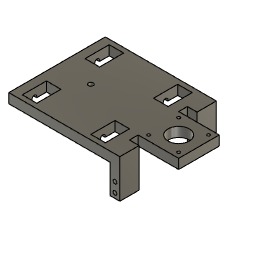
maturita3 v7-asi už konečne final verze (Autodesk Fusion 360 design; units mm, degrees)
Autodesk Fusion 360 part; units mm, degrees
note: some values were not read from the file. Set by a fixed rule: which sketch regions a step uses.
sketch "Sketch1" plane through (0, 0, 0) normal (0, 0, 1) x (1, 0, 0)
  line L0 (0, 0) -> (105, 0)
  line L1 (105, 0) -> (105, 29)
  line L2 (105, 29) -> (147, 29)
  line L3 (147, 29) -> (147, 71)
  line L4 (147, 71) -> (105, 71)
  line L5 (105, 71) -> (105, 100)
  line L6 (105, 100) -> (0, 100)
  line L7 (0, 100) -> (0, 0)
  dimension "d1" = 105
  dimension "d2" = 29
  dimension "d3" = 42
  dimension "d4" = 42
  dimension "d5" = 29
  dimension "d35" = 105
  constraint coincident L0.start L7.end
  constraint horizontal L0
  constraint perpendicular L0 L1
  constraint perpendicular L1 L2
  constraint perpendicular L2 L3
  constraint perpendicular L1 L4
  constraint perpendicular L4 L5
  constraint perpendicular L5 L6
  constraint perpendicular L6 L7
  measures "d1" distance of L0.start L0.end
  measures "d2" distance of L0.end L1.end
  measures "d3" distance of L1.end L2.end
  measures "d4" distance of L2.end L3.end
  measures "d5" distance of L4.end L5.end
  measures "d35" distance of L5.end L6.end
extrude "Extrude1" add sketch "Sketch1" along normal blind 10
sketch "Sketch2" plane through (0, 0, 10) normal (0, 0, 1) x (-1, 0, 0)
  line L0 (0, -100) -> (0, 0)
  line L1 (0, 0) -> (-105, 0)
  line L2 (-105, 0) -> (-105, -29)
  line L3 (-105, -29) -> (-147, -29)
  line L4 (-147, -29) -> (-147, -71)
  line L5 (-147, -71) -> (-105, -71)
  line L6 (-105, -71) -> (-105, -100)
  line L7 (-105, -100) -> (0, -100)
  line L8 (-147, -71) -> (-141.5, -71)
  line L9 (-141.5, -71) -> (-141.5, -65.5)
  line L10 (-141.5, -65.5) -> (-110.5, -65.5)
  line L11 (-110.5, -65.5) -> (-110.5, -34.5)
  line L12 (-110.5, -34.5) -> (-141.5, -34.5)
  line L13 (-141.5, -34.5) -> (-141.5, -65.5)
  dimension "d8" = 5.5
  dimension "d9" = 5.5
  dimension "d10" = 31
  dimension "d11" = 31
  constraint coincident L4.end L5.start
  constraint perpendicular L4 L8
  constraint perpendicular L8 L9
  constraint horizontal L10
  constraint vertical L11
  constraint horizontal L12
  constraint vertical L13
  measures "d8" distance of L4.end L8.end
  measures "d9" distance of L8.end L9.end
  measures "d10" distance of L9.end L10.end
  measures "d11" distance of L9.end L12.end
hole "Hole1" at (110.5, 65.5, 10) at (110.5, 34.5, 10) at (141.5, 34.5, 10) at (141.5, 65.5, 10) direction (0, 0, -1) diameter 3 depth 10 tip angle 180
sketch "Sketch3" plane through (0, 0, 10) normal (0, 0, 1) x (-1, 0, 0)
  circle A0 centre (-141.5, -34.5) radius 1.5
  circle A1 centre (-110.5, -65.5) radius 1.5
  circle A2 centre (-110.5, -34.5) radius 1.5
  circle A3 centre (-141.5, -65.5) radius 1.5
  line L0 (0, -100) -> (0, 0)
  line L1 (0, 0) -> (-105, 0)
  line L2 (-105, 0) -> (-105, -29)
  line L3 (-105, -29) -> (-147, -29)
  line L4 (-147, -29) -> (-147, -71)
  line L5 (-147, -71) -> (-105, -71)
  line L6 (-105, -71) -> (-105, -100)
  line L7 (-105, -100) -> (0, -100)
  line L8 (0, -50) -> (-35, -50)
  circle A4 centre (-35, -50) radius 2.5
  circle A5 centre (-35, -50) radius 5
  dimension "d15" = 5
  dimension "d16" = 10
  dimension "d36" = 35
  constraint midpoint L0 L8.start
  constraint perpendicular L0 L8
  constraint coincident L8.end A4.centre
  measures "d15" diameter of A4
  measures "d16" diameter of A5
  measures "d36" distance of L8.start L8.end
extrude "Extrude2" cut sketch "Sketch3" against normal up to surface (10 mm away) contours A4
extrude "Extrude3" add sketch "Sketch3" along normal blind 1 contours A5
extrude "Extrude4" add 1 faces at (30.8519, 50.2484, 11) along direction (0, 0, -1) blind 20
sketch "Sketch4" plane through (0, 0, -9) normal (0, 0, -1) x (1, 0, 0)
  circle A0 centre (35, -50) radius 2.5
  circle A1 centre (35, -50) radius 5
  circle A2 centre (35, -50) radius 5
  constraint concentric A0 A2
extrude "Extrude5" add sketch "Sketch4" against normal blind 2 contours A0
sketch "Sketch5" plane through (0, 0, 10) normal (0, 0, 1) x (-1, 0, 0)
  line L0 (-115, -100) -> (-95, -100)
  line L1 (-95, -100) -> (-95, -95)
  line L2 (-95, -95) -> (-80, -95)
  line L3 (-80, -95) -> (-80, -70)
  line L4 (-80, -70) -> (-95, -70)
  line L5 (-95, -70) -> (-95, -95)
  dimension "d25" = 20
  dimension "d26" = 5
  dimension "d27" = 15
  dimension "d28" = 25
  constraint horizontal L0
  constraint perpendicular L0 L1
  constraint horizontal L2
  constraint vertical L3
  constraint horizontal L4
  constraint vertical L5
  measures "d25" distance of L0.start L0.end
  measures "d26" distance of L0.end L1.end
  measures "d27" distance of L1.end L2.end
  measures "d28" distance of L1.end L4.end
extrude "Extrude6" cut sketch "Sketch5" against normal blind 10
pattern_linear "R-Pattern1" count 2 spacing 65 along (0, -1, 0) count 2 spacing 71 along (-1, 0, 0) of "Extrude6"
sketch "Sketch6" plane through (0, 0, 10) normal (0, 0, 1) x (-1, 0, 0)
  line L0 (-9, -30) -> (-24, -30)
  line L1 (-24, -30) -> (-24, -5)
  line L2 (-24, -5) -> (-9, -5)
  line L3 (-9, -5) -> (-9, -30)
  line L4 (-9, -95) -> (-24, -95)
  line L5 (-24, -95) -> (-24, -70)
  line L6 (-24, -70) -> (-9, -70)
  line L7 (-9, -70) -> (-9, -95)
  line L8 (-80, -30) -> (-95, -30)
  line L9 (-95, -30) -> (-95, -5)
  line L10 (-95, -5) -> (-80, -5)
  line L11 (-80, -5) -> (-80, -30)
  line L12 (-80, -95) -> (-95, -95)
  line L13 (-95, -95) -> (-95, -70)
  line L14 (-95, -70) -> (-80, -70)
  line L15 (-80, -70) -> (-80, -95)
  circle A0 centre (-35, -50) radius 5
  circle A1 centre (-141.5, -34.5) radius 1.5
  circle A2 centre (-110.5, -65.5) radius 1.5
  circle A3 centre (-110.5, -34.5) radius 1.5
  circle A4 centre (-141.5, -65.5) radius 1.5
  line L16 (0, -100) -> (0, 0)
  line L17 (0, 0) -> (-105, 0)
  line L18 (-105, 0) -> (-105, -29)
  line L19 (-105, -29) -> (-147, -29)
  line L20 (-147, -29) -> (-147, -71)
  line L21 (-147, -71) -> (-105, -71)
  line L22 (-105, -71) -> (-105, -100)
  line L23 (-105, -100) -> (0, -100)
  line L24 (-147, -50) -> (-126, -50)
  constraint midpoint L20 L24.start
  constraint perpendicular L20 L24
hole "Hole2" at (126, 50, 10) direction (0, 0, -1) diameter 22 depth 10 tip angle 180
sketch "Sketch7" plane through (0, 0, 0) normal (0, 0, -1) x (1, 0, 0)
  circle A0 centre (126, -50) radius 11
  line L0 (24, -30) -> (9, -30)
  line L1 (9, -30) -> (9, -5)
  line L2 (9, -5) -> (24, -5)
  line L3 (24, -5) -> (24, -30)
  line L4 (24, -95) -> (9, -95)
  line L5 (9, -95) -> (9, -70)
  line L6 (9, -70) -> (24, -70)
  line L7 (24, -70) -> (24, -95)
  line L8 (95, -30) -> (80, -30)
  line L9 (80, -30) -> (80, -5)
  line L10 (80, -5) -> (95, -5)
  line L11 (95, -5) -> (95, -30)
  line L12 (95, -95) -> (80, -95)
  line L13 (80, -95) -> (80, -70)
  line L14 (80, -70) -> (95, -70)
  line L15 (95, -70) -> (95, -95)
  circle A1 centre (35, -50) radius 5
  circle A2 centre (141.5, -34.5) radius 1.5
  circle A3 centre (110.5, -65.5) radius 1.5
  circle A4 centre (110.5, -34.5) radius 1.5
  circle A5 centre (141.5, -65.5) radius 1.5
  line L16 (0, 0) -> (0, -100)
  line L17 (0, -100) -> (105, -100)
  line L18 (105, -100) -> (105, -71)
  line L19 (105, -71) -> (147, -71)
  line L20 (147, -71) -> (147, -29)
  line L21 (147, -29) -> (105, -29)
  line L22 (105, -29) -> (105, 0)
  line L23 (105, 0) -> (0, 0)
  line L24 (0, -100) -> (50, -100)
  line L25 (50, -100) -> (50, -80)
  line L26 (50, -80) -> (57, -80)
  line L27 (57, -80) -> (57, -60)
  line L28 (57, -60) -> (50, -60)
  line L29 (50, -60) -> (50, -80)
  line L30 (50, -60) -> (50, -40)
  line L31 (50, -40) -> (57, -40)
  line L32 (57, -40) -> (57, -20)
  line L33 (57, -20) -> (50, -20)
  line L34 (50, -20) -> (50, -40)
  dimension "d40" = 50
  dimension "d41" = 20
  dimension "d42" = 7
  dimension "d43" = 20
  dimension "d44" = 20
  dimension "d45" = 7
  dimension "d46" = 20
  constraint coincident L16.end L17.start
  constraint perpendicular L16 L24
  constraint perpendicular L24 L25
  constraint horizontal L26
  constraint vertical L27
  constraint horizontal L28
  constraint vertical L29
  constraint perpendicular L28 L30
  constraint horizontal L31
  constraint vertical L32
  constraint horizontal L33
  constraint vertical L34
  measures "d40" distance of L16.end L24.end
  measures "d41" distance of L24.end L25.end
  measures "d42" distance of L25.end L26.end
  measures "d43" distance of L25.end L28.end
  measures "d44" distance of L28.end L30.end
  measures "d45" distance of L30.end L31.end
  measures "d46" distance of L30.end L33.end
extrude "Extrude7" add sketch "Sketch7" along normal blind 9 contours L26 L27 L28 L29 | L31 L32 L33 L34
sketch "Sketch8" plane through (57, 0, 0) normal (1, 0, 0) x (0, 1, 0)
  line L0 (40, 0) -> (20, 0)
  line L1 (20, 0) -> (20, -9)
  line L2 (20, -9) -> (40, -9)
  line L3 (40, -9) -> (40, 0)
  line L4 (20, -4.5) -> (30, -4.5)
  line L5 (60, -9) -> (70, -9)
  line L6 (70, -9) -> (70, -4.5)
  constraint midpoint L1 L4.start
  constraint perpendicular L1 L4
  constraint horizontal L5
  constraint perpendicular L5 L6
hole "Hole3" at (57, 30, -4.5) at (57, 70, -4.5) direction (-1, 0, 0) diameter 3 depth 10 tip angle 180
sketch "Sketch9" plane through (9, 0, 0) normal (1, 0, 0) x (0, 1, 0)
  line L0 (30, 10) -> (5, 10)
  line L1 (5, 10) -> (5, 0)
  line L2 (5, 0) -> (30, 0)
  line L3 (30, 0) -> (30, 10)
  line L4 (5, 0) -> (17.5, 0)
  line L5 (17.5, 0) -> (17.5, 1)
  circle A0 centre (17.5, 1) radius 2.5
  dimension "d52" = 5
  constraint coincident L1.end L2.start
  constraint midpoint L2 L4.end
  constraint perpendicular L2 L5
  constraint coincident L5.end A0.centre
  measures "d52" diameter of A0
extrude "Extrude8" cut sketch "Sketch9" against normal blind 5 contours L2 L4 A0 | L2 L4 A0
extrude "Extrude9" cut 1 faces at (4, 16.7082, 0.9519) along direction (1, 0, 0) blind 25
pattern_linear "R-Pattern2" count 2 spacing 65 along (0, 1, 0) count 2 spacing 71 along (1, 0, 0) of "Extrude9"
extrude "Extrude10" cut 1 faces at (30.8519, 50.2484, 11) along direction (0, 0, -1) blind 1
sketch "Sketch10" plane through (0, 0, 10) normal (0, 0, 1) x (-1, 0, 0)
  circle A0 centre (-35, -50) radius 2.5
  circle A1 centre (-126, -50) radius 11
  line L0 (-9, -30) -> (-24, -30)
  line L1 (-24, -30) -> (-24, -5)
  line L2 (-24, -5) -> (-9, -5)
  line L3 (-9, -5) -> (-9, -30)
  line L4 (-9, -95) -> (-24, -95)
  line L5 (-24, -95) -> (-24, -70)
  line L6 (-24, -70) -> (-9, -70)
  line L7 (-9, -70) -> (-9, -95)
  line L8 (-80, -30) -> (-95, -30)
  line L9 (-95, -30) -> (-95, -5)
  line L10 (-95, -5) -> (-80, -5)
  line L11 (-80, -5) -> (-80, -30)
  line L12 (-80, -95) -> (-95, -95)
  line L13 (-95, -95) -> (-95, -70)
  line L14 (-95, -70) -> (-80, -70)
  line L15 (-80, -70) -> (-80, -95)
  circle A2 centre (-141.5, -34.5) radius 1.5
  circle A3 centre (-110.5, -65.5) radius 1.5
  circle A4 centre (-110.5, -34.5) radius 1.5
  circle A5 centre (-141.5, -65.5) radius 1.5
  line L16 (0, -100) -> (0, 0)
  line L17 (0, 0) -> (-105, 0)
  line L18 (-105, 0) -> (-105, -29)
  line L19 (-105, -29) -> (-147, -29)
  line L20 (-147, -29) -> (-147, -71)
  line L21 (-147, -71) -> (-105, -71)
  line L22 (-105, -71) -> (-105, -100)
  line L23 (-105, -100) -> (0, -100)
  line L24 (-105, -100) -> (-115, -100)
  line L25 (-115, -100) -> (-115, -80)
  line L26 (-115, -80) -> (-105, -80)
  line L27 (-105, -80) -> (-105, -100)
  line L28 (-105, 0) -> (-115, 0)
  line L29 (-115, 0) -> (-115, -20)
  line L30 (-115, -20) -> (-105, -20)
  line L31 (-105, -20) -> (-105, 0)
  dimension "d63" = 10
  dimension "d64" = 20
  dimension "d65" = 10
  dimension "d66" = 20
  constraint horizontal L24
  constraint vertical L25
  constraint horizontal L26
  constraint vertical L27
  constraint coincident L22.end L23.start
  constraint horizontal L28
  constraint vertical L29
  constraint horizontal L30
  constraint vertical L31
  constraint coincident L17.end L18.start
  measures "d63" distance of L22.end L24.end
  measures "d64" distance of L22.end L26.end
  measures "d65" distance of L17.end L28.end
  measures "d66" distance of L17.end L30.end
extrude "Extrude11" add sketch "Sketch10" against normal blind 40 contours L22 L24 L25 L26 L27 | L18 L28 L29 L30 L31
sketch "Sketch11" plane through (0, 0, 0) normal (0, -1, 0) x (1, 0, 0)
  line L0 (0, 0) -> (105, 0)
  line L1 (105, 0) -> (105, -30)
  line L2 (105, -30) -> (115, -30)
  line L3 (115, -30) -> (115, 10)
  line L4 (115, 10) -> (0, 10)
  line L5 (0, 10) -> (0, 0)
  line L6 (110, -30) -> (110, -25)
  line L7 (110, -25) -> (110, -15)
  dimension "d69" = 5
  dimension "d70" = 10
  constraint midpoint L2 L6.start
  constraint perpendicular L2 L6
  constraint perpendicular L2 L7
  measures "d69" distance of L6.start L6.end
  measures "d70" distance of L6.end L7.end
hole "Hole4" at (110, 0, -25) at (110, 0, -15) direction (0, 1, 0) diameter 4 end through all
equation "d2 = ( ( 100 - 42 ) / 2 ) * 1 mm"
equation "d8 = ( ( 42 - 31 ) / 2 ) * 1 mm"
